Autodesk Fusion 360 part; units mm, degrees
note: some values were not read from the file. Set by a fixed rule: which face or edge a step refers to.
(part 2 of 2)
sketch "Sketch1" plane through (0, 0, 0) normal (0, 0, 1) x (1, 0, 0)
  line L0 (0, 0) -> (72, 0)
  line L1 (72, 0) -> (72, -21)
  line L2 (72, -21) -> (0, -21)
  line L3 (0, -21) -> (0, 0)
  line L4 (0, 0) -> (0, -7)
  line L5 (0, -7) -> (-2, -7)
  line L6 (-2, -7) -> (-2, -14)
  line L7 (-2, -14) -> (0, -14)
  line L8 (0, -14) -> (0, -7)
  line L9 (72, 0) -> (72, -7)
  line L10 (72, -7) -> (74, -7)
  line L11 (74, -7) -> (74, -14)
  line L12 (74, -14) -> (72, -14)
  line L13 (72, -14) -> (72, -7)
  line L14 (72, -21) -> (48, -21)
  line L15 (48, -21) -> (24, -21)
  line L16 (24, -21) -> (24, -23)
  line L17 (24, -23) -> (48, -23)
  line L18 (48, -23) -> (48, -21)
  dimension "d1" = 72
  dimension "d2" = 21
  dimension "d5" = 7
  dimension "d6" = 2
  dimension "d7" = 7
  dimension "d8" = 7
  dimension "d9" = 2
  dimension "d10" = 7
  dimension "d11" = 24
  dimension "d12" = 24
  dimension "d13" = 2
  constraint horizontal L0
  constraint vertical L1
  constraint horizontal L2
  constraint vertical L3
  constraint coincident L0.start L3.end
  constraint perpendicular L0 L4
  constraint horizontal L5
  constraint vertical L6
  constraint horizontal L7
  constraint vertical L8
  constraint perpendicular L0 L9
  constraint horizontal L10
  constraint vertical L11
  constraint horizontal L12
  constraint vertical L13
  constraint perpendicular L1 L14
  constraint horizontal L15
  constraint vertical L16
  constraint horizontal L17
  constraint vertical L18
  measures "d1" distance of L0.start L0.end
  measures "d2" distance of L0.start L2.end
  measures "d5" distance of L0.start L4.end
  measures "d6" distance of L4.end L5.end
  measures "d7" distance of L4.end L7.end
  measures "d8" distance of L0.end L9.end
  measures "d9" distance of L9.end L10.end
  measures "d10" distance of L9.end L12.end
  measures "d11" distance of L1.end L14.end
  measures "d12" distance of L14.end L15.end
  measures "d13" distance of L14.end L17.end
extrude "Extrude1" add sketch "Sketch1" along normal blind 2

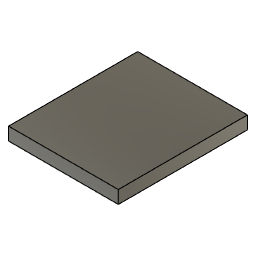
design "PCB_MAIN"
Autodesk Fusion 360 part; units mm, degrees
sketch "Sketch1" plane through (0, 0, 0) normal (0, 0, 1) x (1, 0, 0)
  line L0 (0, 0) -> (68, 0)
  line L1 (68, 0) -> (68, -80)
  line L2 (68, -80) -> (0, -80)
  line L3 (0, -80) -> (0, 0)
  dimension "d1" = 68
  dimension "d2" = 80
  constraint horizontal L0
  constraint vertical L1
  constraint horizontal L2
  constraint vertical L3
  constraint coincident L0.start L3.end
  measures "d1" distance of L0.start L0.end
  measures "d2" distance of L0.start L2.end
extrude "Extrude1" add sketch "Sketch1" along normal blind 8

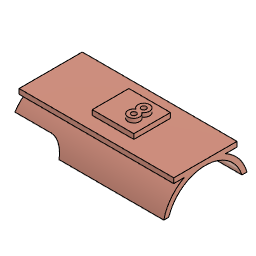
design "Weight_top_old_v2"
Autodesk Fusion 360 part; units mm, degrees
sketch "Sketch1" plane through (0, 0, 0) normal (0, 0, 1) x (1, 0, 0)
  line L0 (93, 0) -> (93, 38)
  line L1 (0, 0) -> (0, 38)
  circle A0 centre (53, 16) radius 1.5
  circle A1 centre (53, 22) radius 1.5
  circle A2 centre (53, 16) radius 2.75
  circle A3 centre (53, 16) radius 3.5
  circle A4 centre (53, 22) radius 2.75
  circle A5 centre (53, 22) radius 3.5
  line L2 (36, 8) -> (61, 8)
  line L3 (61, 8) -> (61, 30)
  line L4 (61, 30) -> (36, 30)
  line L5 (36, 30) -> (36, 8)
  line L6 (0, 38) -> (93, 38)
  line L7 (0, 0) -> (93, 0)
  dimension "d61" = 3
  dimension "d63" = 53
  dimension "d64" = 3
  dimension "d66" = 5.5
  dimension "d67" = 7
  dimension "d68" = 5.5
  dimension "d69" = 7
  dimension "d70" = 25
  dimension "d71" = 22
  dimension "d72" = 32
  dimension "d80" = 93
  constraint vertical L0
  constraint concentric A0 A2
  constraint concentric A2 A3
  constraint concentric A1 A4
  constraint concentric A1 A5
  constraint horizontal L2
  constraint vertical L3
  constraint horizontal L4
  constraint vertical L5
  constraint perpendicular L0 L6
  constraint perpendicular L0 L7
  measures "d61" diameter of A0
  measures "d63" distance of L1 A0.centre
  measures "d64" diameter of A1
  measures "d66" diameter of A2
  measures "d67" diameter of A3
  measures "d68" diameter of A4
  measures "d69" diameter of A5
  measures "d70" distance of L2.start L2.end
  measures "d71" distance of L2.start L4.end
  measures "d72" distance of L0 L3
  measures "d80" distance of L0.end L1.end
extrude "Extrude13" add sketch "Sketch1" along normal blind 3 contours L0 L1 L6 L7 | A2 A3 A5 | A3 A4 A5 | L2 L3 L4 L5
extrude "Extrude14" add sketch "Sketch1" along normal blind 6 contours A0 | A1 | A2 A5 | A2 A3 A5 | A2 A5 | A2 A3 A4 A5 | A3 A4 A5 | A3 A4 | A3 A4 | L2 L3 L4 L5
extrude "Extrude15" add sketch "Sketch1" along normal blind 8.4 contours A0 | A1 | A2 A5 | A2 A3 A5 | A2 A5 | A2 A3 A4 A5 | A3 A4 A5 | A3 A4 | A3 A4
sketch "Sketch3" plane through (0, 0, 0) normal (-1, 0, 0) x (0, -1, 0)
  line L0 (-38, 0) -> (0, 0)
  line L1 (0, 0) -> (0, 3)
  line L2 (0, 3) -> (-38, 3)
  line L3 (-38, 3) -> (-38, 0)
  line L4 (-19, 0) -> (-19, -16)
  arc A0 (-19, 3) -> (-44, -16) centre (-19, -22.9474) ccw
  line L5 (-44, -16) -> (-41, -16)
  arc A1 (-19, 0) -> (-41, -16) centre (-19, -23.125) ccw
  line L6 (-19, -16) -> (3, -16)
  line L7 (3, -16) -> (6, -16)
  line L8 (-19, -16) -> (-41, -16)
  arc A2 (3, -16) -> (-19, 0) centre (-19, -23.125) ccw
  arc A3 (6, -16) -> (-19, 3) centre (-18.0924, -21.7532) ccw
  line L9 (-19, -8) -> (2.5084, -8)
  line L10 (-19, -8) -> (-40.2095, -8)
  dimension "d81" = 16
  dimension "d84" = 3
  dimension "d85" = 22
  dimension "d86" = 3
  dimension "d87" = 22
  constraint midpoint L0 L4.start
  constraint perpendicular L0 L4
  constraint midpoint L2 A0.start
  constraint tangent L0 A1
  constraint perpendicular L4 L6
  constraint parallel L6 L7
  constraint perpendicular L4 L8
  constraint tangent A2 A3
  constraint midpoint L4 L9.start
  constraint coincident A3 L9.end
  constraint perpendicular L4 L9
  constraint coincident A0 L10.end
  constraint perpendicular L4 L10
  measures "d81" distance of L4.start L4.end
  measures "d84" distance of A0.end L5.end
  measures "d85" distance of L4.end L6.end
  measures "d86" distance of L6.end L7.end
  measures "d87" distance of L4.end L5.end
extrude "Extrude16" add sketch "Sketch3" against normal blind 93 contours L0 A0 A1 L10 | L0 A2 A3 L9 | A0 L5 A1 L10 | L7 A2 A3 L9
extrude "Extrude17" cut sketch "Sketch3" against normal blind 30 contours A0 L5 A1 L10 | L7 A2 A3 L9
fillet "Fillet1" radius 8 2 edges at (30, -0.5006, -8) (30, 38.3512, -8)
extrude "Extrude18" cut sketch "Sketch1" along normal blind 2.1 and the other way blind 2.1 contours A0 | A1 | A2 A5 | A2 A5 | A3 A4 | A3 A4
extrude "Extrude19" cut sketch "Sketch1" along normal through all contours A0 | A1

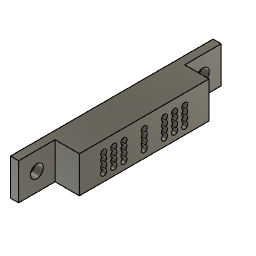
design "Lickport_holder"
Autodesk Fusion 360 part; units mm, degrees
sketch "Sketch1" plane through (0, 0, 0) normal (1, 0, 0) x (0, 1, 0)
  line L0 (0, 0) -> (50, 0)
  line L1 (50, 0) -> (50, -9)
  line L2 (50, -9) -> (0, -9)
  line L3 (0, -9) -> (0, 0)
  circle A0 centre (45.5, -4.5) radius 1.6
  circle A1 centre (4.5, -4.5) radius 1.6
  circle A2 centre (20, -2.8) radius 0.755
  circle A3 centre (32.5, -4.2) radius 0.755
  circle A4 centre (15, -5.6) radius 0.755
  circle A5 centre (15, -4.2) radius 0.755
  circle A6 centre (17.5, -4.2) radius 0.755
  circle A7 centre (30, -2.8) radius 0.755
  circle A8 centre (20, -5.6) radius 0.755
  circle A9 centre (25, -7) radius 0.755
  circle A10 centre (17.5, -2.8) radius 0.755
  circle A11 centre (20, -7) radius 0.755
  circle A12 centre (25, -4.2) radius 0.755
  circle A13 centre (25, -5.6) radius 0.755
  circle A14 centre (32.5, -7) radius 0.755
  circle A15 centre (17.5, -5.6) radius 0.755
  circle A16 centre (30, -4.2) radius 0.755
  circle A17 centre (35, -5.6) radius 0.755
  circle A18 centre (35, -2.8) radius 0.755
  circle A19 centre (30, -7) radius 0.755
  circle A20 centre (20, -4.2) radius 0.755
  circle A21 centre (17.5, -7) radius 0.755
  circle A22 centre (35, -7) radius 0.755
  circle A23 centre (25, -2.8) radius 0.755
  circle A24 centre (32.5, -5.6) radius 0.755
  circle A25 centre (15, -7) radius 0.755
  circle A26 centre (35, -4.2) radius 0.755
  circle A27 centre (30, -5.6) radius 0.755
  circle A28 centre (32.5, -2.8) radius 0.755
  circle A29 centre (15, -2.8) radius 0.755
  line L4 (41, -9) -> (41, 0)
  line L5 (9, -9) -> (9, 0)
  point P0 (25, -2.8)
  point P1 (25, -4.2)
  point P2 (25, -7)
  point P3 (25, -5.6)
  point P4 (25, -2.8)
  dimension "d1" = 50
  dimension "d2" = 9
  dimension "d5" = 3.2
  dimension "d6" = 3.2
  dimension "d7" = 4.5
  dimension "d8" = 4.5
  dimension "d9" = 4.5
  dimension "d10" = 4.5
  dimension "d19" = 1.51
  dimension "d68" = 1.51
  dimension "d70" = 1.51
  dimension "d72" = 10
  dimension "d74" = 1.51
  dimension "d75" = 7.5
  dimension "d169" = 1.51
  dimension "d170" = 1.51
  dimension "d171" = 1.51
  dimension "d172" = 1.51
  dimension "d173" = 1.51
  dimension "d174" = 10
  dimension "d175" = 10
  dimension "d176" = 1.51
  dimension "d177" = 1.51
  dimension "d178" = 7.5
  dimension "d179" = 7.5
  dimension "d181" = 1.51
  dimension "d183" = 1.51
  dimension "d185" = 10
  dimension "d187" = 1.51
  dimension "d190" = 7.5
  dimension "d191" = 1.51
  dimension "d192" = 1.51
  dimension "d193" = 1.51
  dimension "d194" = 1.51
  dimension "d195" = 1.51
  dimension "d196" = 10
  dimension "d197" = 10
  dimension "d198" = 1.51
  dimension "d199" = 1.51
  dimension "d200" = 7.5
  dimension "d201" = 7.5
  dimension "d202" = 1.51
  dimension "d203" = 1.51
  dimension "d204" = 1.51
  dimension "d205" = 1.51
  dimension "d206" = 1.51
  dimension "d207" = 10
  dimension "d208" = 10
  dimension "d209" = 1.51
  dimension "d210" = 1.51
  dimension "d211" = 7.5
  dimension "d212" = 7.5
  dimension "d78" = 9
  dimension "d79" = 9
  constraint horizontal L0
  constraint vertical L1
  constraint horizontal L2
  constraint vertical L3
  constraint coincident L0.start L3.end
  constraint coincident P4 P0
  constraint coincident P1 A12.centre
  constraint coincident P3 A13.centre
  constraint coincident P2 A9.centre
  constraint coincident L2 L4.start
  constraint coincident L0 L4.end
  constraint perpendicular L0 L4
  constraint coincident L2 L5.start
  constraint coincident L0 L5.end
  constraint perpendicular L0 L5
  measures "d1" distance of L0.start L0.end
  measures "d2" distance of L0.start L2.end
  measures "d5" diameter of A0
  measures "d6" diameter of A1
  measures "d7" distance of L2 A0.centre
  measures "d8" distance of L1 A0.centre
  measures "d9" distance of L3 A1.centre
  measures "d10" distance of L2 A1.centre
  measures "d19" diameter of A2
  measures "d68" diameter of A23
  measures "d70" diameter of A29
  measures "d72" distance of P4 A29.centre
  measures "d74" diameter of A10
  measures "d75" distance of A10.centre P4
  measures "d169" diameter of A20
  measures "d170" diameter of A16
  measures "d171" diameter of A12
  measures "d172" diameter of A26
  measures "d173" diameter of A5
  measures "d174" distance of P1 A26.centre
  measures "d175" distance of P1 A5.centre
  measures "d176" diameter of A3
  measures "d177" diameter of A6
  measures "d178" distance of P1 A6.centre
  measures "d179" distance of P1 A3.centre
  measures "d181" diameter of A7
  measures "d183" diameter of A18
  measures "d185" distance of P4 A18.centre
  measures "d187" diameter of A28
  measures "d190" distance of P4 A28.centre
  measures "d191" diameter of A8
  measures "d192" diameter of A27
  measures "d193" diameter of A13
  measures "d194" diameter of A17
  measures "d195" diameter of A4
  measures "d196" distance of P3 A17.centre
  measures "d197" distance of P3 A4.centre
  measures "d198" diameter of A24
  measures "d199" diameter of A15
  measures "d200" distance of P3 A15.centre
  measures "d201" distance of P3 A24.centre
  measures "d202" diameter of A11
  measures "d203" diameter of A19
  measures "d204" diameter of A9
  measures "d205" diameter of A22
  measures "d206" diameter of A25
  measures "d207" distance of P2 A22.centre
  measures "d208" distance of P2 A25.centre
  measures "d209" diameter of A14
  measures "d210" diameter of A21
  measures "d211" distance of P2 A21.centre
  measures "d212" distance of P2 A14.centre
  measures "d78" distance of L1 L4
  measures "d79" distance of L3 L5
extrude "Extrude1" add sketch "Sketch1" along normal blind 8 contours L0 L2 L4 L5
extrude "Extrude2" add sketch "Sketch1" along normal blind 2 contours L0 L2 L3 L5 | L0 L1 L2 L4

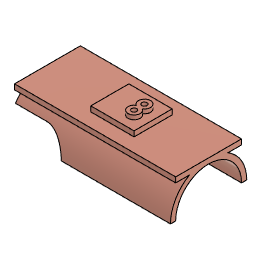
design "Weight_top"
Autodesk Fusion 360 part; units mm, degrees
sketch "Sketch1" plane through (0, 0, 0) normal (0, 0, 1) x (1, 0, 0)
  line L0 (93, 0) -> (93, 38)
  line L1 (0, 0) -> (0, 38)
  circle A0 centre (53, 16) radius 1.5
  circle A1 centre (53, 22) radius 1.5
  circle A2 centre (53, 16) radius 2.75
  circle A3 centre (53, 16) radius 3.5
  circle A4 centre (53, 22) radius 2.75
  circle A5 centre (53, 22) radius 3.5
  line L2 (36, 8) -> (61, 8)
  line L3 (61, 8) -> (61, 30)
  line L4 (61, 30) -> (36, 30)
  line L5 (36, 30) -> (36, 8)
  line L6 (0, 38) -> (93, 38)
  line L7 (0, 0) -> (93, 0)
  dimension "d61" = 3
  dimension "d63" = 53
  dimension "d64" = 3
  dimension "d66" = 5.5
  dimension "d67" = 7
  dimension "d68" = 5.5
  dimension "d69" = 7
  dimension "d70" = 25
  dimension "d71" = 22
  dimension "d72" = 32
  dimension "d80" = 93
  constraint vertical L0
  constraint concentric A0 A2
  constraint concentric A2 A3
  constraint concentric A1 A4
  constraint concentric A1 A5
  constraint horizontal L2
  constraint vertical L3
  constraint horizontal L4
  constraint vertical L5
  constraint perpendicular L0 L6
  constraint perpendicular L0 L7
  measures "d61" diameter of A0
  measures "d63" distance of L1 A0.centre
  measures "d64" diameter of A1
  measures "d66" diameter of A2
  measures "d67" diameter of A3
  measures "d68" diameter of A4
  measures "d69" diameter of A5
  measures "d70" distance of L2.start L2.end
  measures "d71" distance of L2.start L4.end
  measures "d72" distance of L0 L3
  measures "d80" distance of L0.end L1.end
extrude "Extrude13" add sketch "Sketch1" along normal blind 3 contours L0 L1 L6 L7 | A2 A3 A5 | A3 A4 A5 | L2 L3 L4 L5
extrude "Extrude14" add sketch "Sketch1" along normal blind 6 contours A0 | A1 | A2 A5 | A2 A3 A5 | A2 A5 | A2 A3 A4 A5 | A3 A4 A5 | A3 A4 | A3 A4 | L2 L3 L4 L5
extrude "Extrude15" add sketch "Sketch1" along normal blind 8.4 contours A0 | A1 | A2 A5 | A2 A3 A5 | A2 A5 | A2 A3 A4 A5 | A3 A4 A5 | A3 A4 | A3 A4
sketch "Sketch3" plane through (0, 0, 0) normal (-1, 0, 0) x (0, -1, 0)
  line L0 (-38, 0) -> (0, 0)
  line L1 (0, 0) -> (0, 3)
  line L2 (0, 3) -> (-38, 3)
  line L3 (-38, 3) -> (-38, 0)
  line L4 (-19, -19) -> (0, -19)
  line L5 (0, -19) -> (3, -19)
  line L6 (-19, -19) -> (-38, -19)
  arc A0 (0, -19) -> (-19, 0) centre (-19, -19) ccw
  arc A1 (3, -19) -> (-19, 3) centre (-19, -19) ccw
  arc A2 (-19, 0) -> (-38, -19) centre (-19, -19) ccw
  line L7 (-38, -19) -> (-41, -19)
  arc A3 (-19, 3) -> (-41, -19) centre (-19, -19) ccw
  line L8 (-19, 0) -> (-19, -7)
  line L9 (-19, -7) -> (-33.7309, -7)
  line L10 (-33.7309, -7) -> (-37.4391, -7)
  line L11 (-19, -7) -> (-4.2691, -7)
  line L12 (-4.2691, -7) -> (-0.5609, -7)
  dimension "d81" = 19
  dimension "d85" = 19
  dimension "d86" = 3
  dimension "d87" = 19
  dimension "d99" = 3
  dimension "d109" = 7
  constraint midpoint L0 A0.end
  constraint parallel L4 L5
  constraint tangent L0 A0
  constraint tangent L2 A1
  constraint midpoint L2 A1.end
  constraint tangent L0 A2
  constraint horizontal L7
  constraint tangent L2 A3
  constraint perpendicular L6 L8
  constraint coincident A2 L9.end
  constraint perpendicular L8 L9
  constraint coincident A3 L10.end
  constraint parallel L9 L10
  constraint coincident A0 L11.end
  constraint perpendicular L8 L11
  constraint coincident A1 L12.end
  constraint parallel L11 L12
  measures "d81" distance of A0.end L4.start
  measures "d85" distance of L4.start L4.end
  measures "d86" distance of L4.end L5.end
  measures "d87" distance of L4.start L6.end
  measures "d99" distance of L6.end L7.end
  measures "d109" distance of A0.end L8.end
extrude "Extrude16" add sketch "Sketch3" against normal blind 93 contours L0 A1 A3 | L0 A2 A3 L10 | L0 A0 A1 L12 | A2 L7 A3 L10 | L5 A0 A1 L12
extrude "Extrude18" cut sketch "Sketch1" along normal blind 2.1 and the other way blind 2.1 contours A0 | A1 | A2 A5 | A2 A5 | A3 A4 | A3 A4
extrude "Extrude19" cut sketch "Sketch1" along normal through all contours A0 | A1
sketch "Sketch4" plane through (93, 0, 0) normal (1, 0, 0) x (0, 1, 0)
  line L0 (0, 0) -> (7.9095, 0)
  arc A0 (7.9095, 0) -> (-3, -19) centre (19, -19) ccw
  line L1 (-3, -19) -> (0, -19)
  arc A1 (38, -19) -> (0, -19) centre (19, -19) ccw
  line L2 (38, -19) -> (41, -19)
  arc A2 (41, -19) -> (30.0905, 0) centre (19, -19) ccw
  line L3 (30.0905, 0) -> (38, 0)
  line L4 (38, 0) -> (38, 3)
  line L5 (38, 3) -> (0, 3)
  line L6 (0, 3) -> (0, 0)
  line L7 (19, -19) -> (-3, -19)
  line L8 (-3, -19) -> (-6, -19)
  line L9 (19, -19) -> (41, -19)
  line L10 (41, -19) -> (44, -19)
  arc A3 (38, -19) -> (-3, -19) centre (17.5, -19) ccw
  arc A4 (44, -19) -> (19, 3) centre (19, -22.2045) ccw
  arc A5 (41, -19) -> (38, -19) centre (39.5, -109.6578) ccw
  arc A6 (19, 3) -> (-6, -19) centre (19, -22.2045) ccw
  line L11 (38, -19) -> (38, -26)
  line L12 (38, -26) -> (74.4637, -26)
  line L13 (74.4637, -26) -> (43.9171, -26)
  line L14 (38, -26) -> (-1.7678, -26)
  line L15 (-5.9171, -26) -> (-1.7678, -26)
  dimension "d100" = 3
  dimension "d101" = 3
  dimension "d102" = 22
  dimension "d103" = 22
  dimension "d105" = 7
  constraint coincident A0.centre A1.centre
  constraint coincident A0.end L1.start
  constraint parallel L7 L8
  constraint coincident L2.end A2.start
  constraint parallel L9 L10
  constraint tangent A1 A3
  constraint coincident A1.start L2.start
  constraint midpoint L5 A4.end
  constraint vertical L11
  constraint coincident A5 L12.end
  constraint perpendicular L11 L12
  constraint coincident A4 L13.end
  constraint horizontal L13
  constraint coincident A3 L14.end
  constraint perpendicular L11 L14
  constraint coincident A6 L15.start
  constraint horizontal L15
  measures "d100" distance of A0.end L8.end
  measures "d101" distance of L2.end L10.end
  measures "d102" distance of A0.centre L2.end
  measures "d103" distance of A0.centre A0.end
  measures "d105" distance of A1.start L11.end
extrude "Extrude21" cut sketch "Sketch3" against normal blind 30 contours A2 L7 A3 L10 | L5 A0 A1 L12
fillet "Fillet2" radius 12 2 edges at (30, 2.415, -7) (30, 35.585, -7)

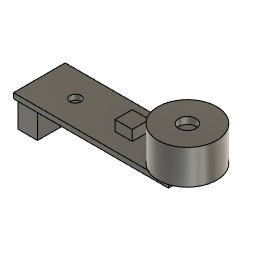
design "PCB_LRT"
Autodesk Fusion 360 part; units mm, degrees
sketch "Sketch1" plane through (0, 0, 0) normal (0, 0, 1) x (1, 0, 0)
  line L0 (0, 0) -> (45, 0)
  line L1 (45, 0) -> (45, -15)
  line L2 (45, -15) -> (0, -15)
  line L3 (0, -15) -> (0, 0)
  line L4 (0, 0) -> (6, 0)
  line L5 (6, 0) -> (6, -15)
  line L6 (6, -15) -> (0, -15)
  line L7 (0, -15) -> (0, 0)
  circle A0 centre (10.5, -7.5) radius 1.6
  circle A1 centre (43, -7.5) radius 8.5
  line L8 (0.3369, -14.0209) -> (6, -14.0209)
  line L9 (6, -14.0209) -> (6, -1)
  line L10 (6, -1) -> (0.3369, -1)
  line L11 (0.3369, -1) -> (0.3369, -14.0209)
  line L12 (29.5, -10) -> (24.5, -10)
  line L13 (24.5, -10) -> (24.5, -5)
  line L14 (24.5, -5) -> (29.5, -5)
  line L15 (29.5, -5) -> (29.5, -10)
  line L16 (29.5, -10) -> (24.5, -5) construction
  line L17 (24.5, -10) -> (29.5, -5) construction
  circle A2 centre (43, -7.5) radius 2.5
  point P0 (27, -7.5)
  point P1 (27, -7.5)
  dimension "d1" = 45
  dimension "d2" = 15
  dimension "d3" = 6
  dimension "d4" = 3.2
  dimension "d5" = 4.5
  dimension "d6" = 17
  dimension "d7" = 43
  dimension "d20" = 27
  dimension "d21" = 5
  dimension "d22" = 5
  constraint horizontal L0
  constraint vertical L1
  constraint horizontal L2
  constraint vertical L3
  constraint coincident L0.start L3.end
  constraint horizontal L4
  constraint vertical L5
  constraint horizontal L6
  constraint vertical L7
  constraint horizontal L8
  constraint vertical L9
  constraint horizontal L10
  constraint vertical L11
  constraint horizontal L12
  constraint perpendicular L12 L13
  constraint parallel L12 L14
  constraint parallel L13 L15
  constraint coincident L16 P1
  constraint coincident L17 P1
  constraint coincident P1 P0
  constraint concentric A1 A2
  measures "d1" distance of L0.start L0.end
  measures "d2" distance of L0.start L2.end
  measures "d3" distance of L0.start L4.end
  measures "d4" diameter of A0
  measures "d5" distance of L5 A0.centre
  measures "d6" diameter of A1
  measures "d7" distance of L3 A1.centre
  measures "d20" distance of L7 P1
  measures "d21" distance of L13.end L14.end
  measures "d22" distance of L12.end L13.end
extrude "Extrude1" add sketch "Sketch1" along normal blind 1.5 contours L0 L2 L3 L4 L5 L6 L7 L8 L10 L11 | L0 L2 L5 A1 L9 | L0 L1 L2 A1 A2 | L5 L8 L9 L10 L11 | L1 A2 | L12 L13 L14 L15 picked at (42.249, -13.3291) picked at (42.7068, -6.9293) makes body 1
extrude "Extrude2" add sketch "Sketch1" along normal blind 10 from surface at 1.5 separate body contours L0 L1 L2 A1 A2 | L0 L1 L2 A1 A2 | L1 A2 | L1 A2 makes body 2
extrude "Extrude4" add sketch "Sketch1" against normal blind 8 contours L5 L8 L9 L10 L11 bodies 1
extrude "Extrude5" add sketch "Sketch1" along normal blind 3 from surface at 1.5 separate body contours L12 L13 L14 L15 makes body 3
extrude "Extrude6" cut sketch "Sketch1" against normal blind 2 from surface at 11.5 contours L1 A2 | L1 A2 bodies 2

design "tray_back_205x55_trans_3mm"
Autodesk Fusion 360 part; units mm, degrees
sketch "Sketch1" plane through (0, 0, 0) normal (0, 0, 1) x (1, 0, 0)
  line L0 (0, 0) -> (200, 0)
  line L1 (200, 0) -> (200, -55)
  line L2 (200, -55) -> (0, -55)
  line L3 (0, -55) -> (0, 0)
  line L4 (0, -55) -> (3.5, -55)
  line L5 (3.5, -55) -> (3.5, -38)
  line L6 (3.5, -38) -> (0, -38)
  line L7 (0, -38) -> (0, -55)
  line L8 (3.5, -38) -> (5.6, -38)
  line L9 (5.6, -38) -> (5.6, -27.8)
  line L10 (5.6, -27.8) -> (3.5, -27.8)
  line L11 (3.5, -27.8) -> (3.5, -38)
  line L12 (200, -55) -> (196.5, -55)
  line L13 (196.5, -55) -> (196.5, -38)
  line L14 (196.5, -38) -> (200, -38)
  line L15 (200, -38) -> (200, -55)
  line L16 (196.5, -38) -> (194.4, -38)
  line L17 (194.4, -38) -> (194.4, -27.8)
  line L18 (194.4, -27.8) -> (196.5, -27.8)
  line L19 (196.5, -27.8) -> (196.5, -38)
  line L20 (196.5, -55) -> (146.5, -55)
  line L21 (146.5, -55) -> (146.5, -50)
  line L22 (146.5, -50) -> (116.3, -50)
  line L23 (116.3, -50) -> (116.3, -47.9)
  line L24 (116.3, -47.9) -> (146.5, -47.9)
  line L25 (146.5, -47.9) -> (146.5, -50)
  line L26 (116.3, -50) -> (66.3, -50)
  line L27 (66.3, -50) -> (36.1, -50)
  line L28 (36.1, -50) -> (36.1, -47.9)
  line L29 (36.1, -47.9) -> (66.3, -47.9)
  line L30 (66.3, -47.9) -> (66.3, -50)
  dimension "d1" = 200
  dimension "d2" = 55
  dimension "d5" = 3.5
  dimension "d6" = 17
  dimension "d7" = 2.1
  dimension "d8" = 10.2
  dimension "d9" = 3.5
  dimension "d10" = 17
  dimension "d11" = 2.1
  dimension "d12" = 10.2
  dimension "d13" = 50
  dimension "d14" = 5
  dimension "d15" = 30.2
  dimension "d16" = 2.1
  dimension "d17" = 50
  dimension "d18" = 30.2
  dimension "d19" = 2.1
  constraint horizontal L0
  constraint vertical L1
  constraint horizontal L2
  constraint vertical L3
  constraint coincident L0.start L3.end
  constraint horizontal L4
  constraint vertical L5
  constraint horizontal L6
  constraint vertical L7
  constraint horizontal L8
  constraint vertical L9
  constraint horizontal L10
  constraint vertical L11
  constraint horizontal L12
  constraint vertical L13
  constraint horizontal L14
  constraint vertical L15
  constraint horizontal L16
  constraint vertical L17
  constraint horizontal L18
  constraint vertical L19
  constraint perpendicular L13 L20
  constraint perpendicular L2 L21
  constraint horizontal L22
  constraint vertical L23
  constraint horizontal L24
  constraint vertical L25
  constraint perpendicular L23 L26
  constraint horizontal L27
  constraint vertical L28
  constraint horizontal L29
  constraint vertical L30
  measures "d1" distance of L0.start L0.end
  measures "d2" distance of L0.start L2.end
  measures "d5" distance of L2.end L4.end
  measures "d6" distance of L2.end L6.end
  measures "d7" distance of L5.end L8.end
  measures "d8" distance of L5.end L10.end
  measures "d9" distance of L1.end L12.end
  measures "d10" distance of L1.end L14.end
  measures "d11" distance of L13.end L16.end
  measures "d12" distance of L13.end L18.end
  measures "d13" distance of L12.end L20.end
  measures "d14" distance of L20.end L21.end
  measures "d15" distance of L21.end L22.end
  measures "d16" distance of L21.end L24.end
  measures "d17" distance of L22.end L26.end
  measures "d18" distance of L26.end L27.end
  measures "d19" distance of L26.end L29.end
extrude "Extrude1" add sketch "Sketch1" along normal blind 3
extrude "Extrude2" add 2 faces at (200, -43.6667, 1) (200, -12.6667, 1) along direction (1, 0, 0) blind 2.5
extrude "Extrude3" add 1 faces at (0, -36.6667, 1) along direction (-1, 0, 0) blind 2.5

design "Weight_top_old_v1"
Autodesk Fusion 360 part; units mm, degrees
sketch "Sketch1" plane through (0, 0, 0) normal (0, 0, 1) x (1, 0, 0)
  line L0 (0, 0) -> (75, 0)
  line L1 (75, 0) -> (75, -50)
  line L2 (75, -50) -> (0, -50)
  line L3 (0, -50) -> (0, 0)
  circle A0 centre (55, -22) radius 1.5
  circle A1 centre (55, -28) radius 1.5
  circle A2 centre (55, -22) radius 2.75
  circle A3 centre (55, -22) radius 3.5
  circle A4 centre (55, -28) radius 2.75
  circle A5 centre (55, -28) radius 3.5
  line L4 (38, -14) -> (63, -14)
  line L5 (63, -14) -> (63, -36)
  line L6 (63, -36) -> (38, -36)
  line L7 (38, -36) -> (38, -14)
  dimension "d1" = 75
  dimension "d2" = 50
  dimension "d3" = 3
  dimension "d4" = 3
  dimension "d5" = 22
  dimension "d6" = 22
  dimension "d7" = 55
  dimension "d8" = 55
  dimension "d9" = 5.5
  dimension "d10" = 7
  dimension "d11" = 5.5
  dimension "d12" = 7
  dimension "d13" = 25
  dimension "d14" = 22
  dimension "d15" = 14
  dimension "d16" = 12
  constraint horizontal L0
  constraint vertical L1
  constraint horizontal L2
  constraint vertical L3
  constraint coincident L0.start L3.end
  constraint concentric A0 A2
  constraint concentric A0 A3
  constraint concentric A1 A4
  constraint concentric A4 A5
  constraint horizontal L4
  constraint vertical L5
  constraint horizontal L6
  constraint vertical L7
  measures "d1" distance of L0.start L0.end
  measures "d2" distance of L0.start L2.end
  measures "d3" diameter of A0
  measures "d4" diameter of A1
  measures "d5" distance of L0 A0.centre
  measures "d6" distance of L2 A1.centre
  measures "d7" distance of L3 A0.centre
  measures "d8" distance of L3 A1.centre
  measures "d9" diameter of A2
  measures "d10" diameter of A3
  measures "d11" diameter of A4
  measures "d12" diameter of A5
  measures "d13" distance of L4.start L4.end
  measures "d14" distance of L4.start L6.end
  measures "d15" distance of L0 L4
  measures "d16" distance of L1 L5
extrude "Extrude1" add sketch "Sketch1" along normal blind 3 contours L0 L1 L2 L3
extrude "Extrude2" add sketch "Sketch1" along normal blind 6 contours L4 L5 L6 L7
extrude "Extrude3" add sketch "Sketch1" along normal blind 8.4 contours A2 A5 | A2 A3 A5 | A2 A5 | A2 A3 A4 A5 | A3 A4 A5 | A3 A4 | A3 A4
sketch "Sketch2" plane through (75, 0, 0) normal (1, 0, 0) x (0, 1, 0)
  line L0 (-50, 0) -> (0, 0)
  line L1 (0, 0) -> (0, 3)
  line L2 (0, 3) -> (-50, 3)
  line L3 (-50, 3) -> (-50, 0)
  line L4 (-25, 3) -> (-25, -16)
  circle A0 centre (-25, -16) radius 19
  circle A1 centre (-25, -16) radius 16
  line L5 (-25, -16) -> (-44, -16)
  line L6 (-25, -16) -> (-6, -16)
  line L7 (-25, -16) -> (-25, -8)
  line L8 (-25, -8) -> (-7.7663, -8)
  line L9 (-25, -8) -> (-42.2337, -8)
  dimension "d23" = 19
  constraint midpoint L2 L4.start
  constraint perpendicular L0 L4
  constraint coincident L4.end A0.centre
  constraint coincident L4.start A0
  constraint concentric A0 A1
  constraint tangent L0 A1
  constraint coincident A0 L5.end
  constraint perpendicular L4 L5
  constraint coincident A0 L6.end
  constraint parallel L5 L6
  constraint coincident L4 L7.end
  constraint perpendicular L6 L7
  constraint coincident A0 L8.end
  constraint perpendicular L4 L8
  constraint coincident A0 L9.end
  constraint perpendicular L4 L9
  measures "d23" distance of L4.start L4.end
extrude "Extrude4" add sketch "Sketch2" against normal blind 75 contours L0 L4 A0 | L0 A0 A1 L9 | L0 L4 A0 | L0 A0 A1 L8 | A0 A1 L5 L9 | A0 A1 L6 L8
extrude "Extrude5" cut sketch "Sketch1" along normal blind -5 and the other way blind -5 contours A0 | A1
extrude "Extrude6" cut sketch "Sketch1" along normal blind -2.1 and the other way blind -2.1 contours A2 A5 | A2 A5 | A3 A4 | A3 A4
extrude "Extrude8" cut 1 faces at (50, -50, 1) along direction (0, 1, 0) blind 6
extrude "Extrude10" cut 1 faces at (25, 0, 1) along direction (0, -1, 0) blind 6
extrude "Extrude11" cut 1 faces at (0, -28.4157, 2) along direction (1, 0, 0) blind 2
extrude "Extrude12" cut sketch "Sketch2" along normal blind 20 from surface at -73 contours A0 A1 L5 L9 | A0 A1 L6 L8

design "cage_top_screw_holder"
Autodesk Fusion 360 part; units mm, degrees
sketch "Sketch1" plane through (0, 0, 0) normal (0, 0, 1) x (1, 0, 0)
  line L0 (0, 0) -> (17.5, 0)
  line L1 (17.5, 0) -> (17.5, -7)
  line L2 (17.5, -7) -> (0, -7)
  line L3 (0, -7) -> (0, 0)
  circle A0 centre (3.75, -3.5) radius 1.25
  circle A1 centre (13.75, -3.5) radius 1.25
  dimension "d1" = 17.5
  dimension "d2" = 7
  dimension "d3" = 2.5
  dimension "d4" = 2.5
  dimension "d5" = 3.75
  dimension "d6" = 3.75
  constraint horizontal L0
  constraint vertical L1
  constraint horizontal L2
  constraint vertical L3
  constraint coincident L0.start L3.end
  measures "d1" distance of L0.start L0.end
  measures "d2" distance of L0.start L2.end
  measures "d3" diameter of A0
  measures "d4" diameter of A1
  measures "d5" distance of L3 A0.centre
  measures "d6" distance of L1 A1.centre
extrude "Extrude1" add sketch "Sketch1" along normal blind 8
sketch "Sketch2" plane through (0, -7, 0) normal (0, -1, 0) x (1, 0, 0)
  line L0 (0, 0) -> (17.5, 0)
  line L1 (17.5, 0) -> (17.5, 8)
  line L2 (17.5, 8) -> (0, 8)
  line L3 (0, 8) -> (0, 0)
  circle A0 centre (8.75, 4) radius 1.25
  dimension "d9" = 2.5
  dimension "d10" = 8.75
  measures "d9" diameter of A0
  measures "d10" distance of L3 A0.centre
extrude "Extrude2" cut sketch "Sketch2" against normal blind 7 contours A0

design "cage_top_310x210_blk_3mm"
Autodesk Fusion 360 part; units mm, degrees
sketch "Sketch1" plane through (0, 0, 0) normal (0, 0, 1) x (1, 0, 0)
  line L0 (0, 0) -> (310, 0)
  line L1 (310, 0) -> (310, -210)
  line L2 (310, -210) -> (0, -210)
  line L3 (0, -210) -> (0, 0)
  circle A0 centre (156.0901, -105) radius 7.05
  circle A1 centre (306.5, -110) radius 1.6
  circle A2 centre (306.5, -100) radius 1.6
  dimension "d1" = 310
  dimension "d2" = 210
  dimension "d9" = 14.1
  dimension "d37" = 3.2
  dimension "d39" = 3.2
  dimension "d41" = 3.5
  dimension "d42" = 3.5
  dimension "d43" = 10
  dimension "d42" = 3.5
  constraint horizontal L0
  constraint vertical L1
  constraint horizontal L2
  constraint vertical L3
  constraint coincident L0.start L3.end
  measures "d1" distance of L0.start L0.end
  measures "d2" distance of L0.start L2.end
  measures "d9" diameter of A0
  measures "d37" diameter of A1
  measures "d39" diameter of A2
  measures "d41" distance of L1 A1.centre
  measures "d42" distance of L1 A2.centre
  measures "d43" distance of A1.centre A2.centre
extrude "Extrude1" add sketch "Sketch1" along normal blind 3

design "weight_bottom"
Autodesk Fusion 360 part; units mm, degrees
sketch "Sketch1" plane through (0, 0, 0) normal (0, 0, 1) x (1, 0, 0)
  line L0 (15, -22) -> (15, -28)
  circle A0 centre (15, -22) radius 3.5
  circle A1 centre (15, -22) radius 1.6
  circle A2 centre (15, -28) radius 3.5
  circle A3 centre (15, -28) radius 1.6
  circle A4 centre (15, -22) radius 2.75
  circle A5 centre (15, -28) radius 2.75
  line L1 (0, -35) -> (2, -35)
  line L2 (2, -35) -> (22, -35)
  line L3 (22, -35) -> (22, -15)
  line L4 (0, -15) -> (0, -35)
  line L5 (7, -15) -> (7, -35)
  line L6 (0, -15) -> (22, -15)
  dimension "d5" = 6
  dimension "d6" = 7
  dimension "d7" = 3.2
  dimension "d8" = 7
  dimension "d9" = 3.2
  dimension "d10" = 5.5
  dimension "d11" = 5.5
  dimension "d65" = 7
  dimension "d66" = 20
  constraint coincident L0.start A0.centre
  constraint concentric A0 A1
  constraint coincident L0.end A2.centre
  constraint concentric A2 A3
  constraint concentric A1 A4
  constraint concentric A2 A5
  constraint perpendicular L2 L3
  constraint perpendicular L1 L4
  constraint coincident L2 L5.end
  constraint perpendicular L2 L5
  measures "d5" distance of L0.start L0.end
  measures "d6" diameter of A0
  measures "d7" diameter of A1
  measures "d8" diameter of A2
  measures "d9" diameter of A3
  measures "d10" diameter of A4
  measures "d11" diameter of A5
  measures "d65" distance of L4 L5
  measures "d66" distance of L4.start L1.start
extrude "Extrude15" add sketch "Sketch1" along normal blind 5 contours L2 L3 L5 L6
extrude "Extrude16" add sketch "Sketch1" along normal blind 15 contours L1 L2 L4 L5 L6
extrude "Extrude17" add sketch "Sketch1" along normal blind 8.4 contours L0 A2 A4 | A2 A4 | L0 A2 A4 | L0 A0 A2 A4 A5 | L0 A0 A2 A4 A5 | A0 A2 A4 | L0 A0 A5 | L0 A0 A5 | A0 A2 A5 | A0 A5
sketch "Sketch5" plane through (7, 0, 0) normal (1, 0, 0) x (0, 1, 0)
  line L0 (-35, 5) -> (-15, 5)
  line L1 (-15, 15) -> (-35, 15)
  line L2 (-35, 15) -> (-35, 5)
  circle A0 centre (-25, 11) radius 2.5
  circle A1 centre (-18, 10) radius 1.25
  circle A2 centre (-32, 10) radius 1.25
  line L3 (-15, 5) -> (-15, 15)
  dimension "d77" = 5
  dimension "d78" = 2.5
  dimension "d79" = 2.5
  dimension "d91" = 4
  dimension "d92" = 5
  dimension "d93" = 5
  measures "d77" diameter of A0
  measures "d78" diameter of A1
  measures "d79" diameter of A2
  measures "d91" distance of L1 A0.centre
  measures "d92" distance of L1 A2.centre
  measures "d93" distance of L1 A1.centre
extrude "Extrude19" cut sketch "Sketch5" against normal blind 7 contours A0 | A1 | A2
extrude "Extrude20" add 1 faces at (8.5111, -25.8394, 5) along direction (0, 0, 1) blind 2.5
extrude "Extrude21" cut 1 faces at (4.4904, -24.1572, 0) along direction (0, 0, 1) blind 2.5
extrude "Extrude22" cut sketch "Sketch1" along normal blind 2 from surface at 2.5 contours L0 A2 A4 | A2 A4 | L0 A2 A4 | L0 A0 A5 | L0 A0 A5 | A0 A5

design "Tube"
Autodesk Fusion 360 part; units mm, degrees
sketch "Sketch1" plane through (0, 0, 0) normal (0, 0, 1) x (1, 0, 0)
  circle A0 centre (0, 0) radius 15
  circle A1 centre (0, 0) radius 2.5
  circle A2 centre (0, 0) radius 17.5
  dimension "d1" = 30
  dimension "d2" = 5
  dimension "d3" = 35
  constraint coincident A0.centre A1.centre
  constraint concentric A0 A1
  constraint concentric A0 A2
  measures "d1" diameter of A0
  measures "d2" diameter of A1
  measures "d3" diameter of A2
extrude "Extrude1" add sketch "Sketch1" along normal blind 100 from surface at 18 contours A0 | A1
loft "Loft1" add profiles "Sketch1" section 1 contours A1 section 2 face at (0.9463, -5.6032, 18)
extrude "Extrude2" add sketch "Sketch1" along normal blind 12 from surface at 106 contours A2
fillet "Fillet1" radius 2.5 1 edges at (-13.9849, -5.4242, 18)
fillet "Fillet2" radius 1 1 edges at (-2.3308, -0.904, 0)
fillet "Fillet3" radius 1 1 edges at (-16.3157, -6.3283, 118)
fillet "Fillet4" radius 1 1 edges at (-16.3157, -6.3283, 106)
